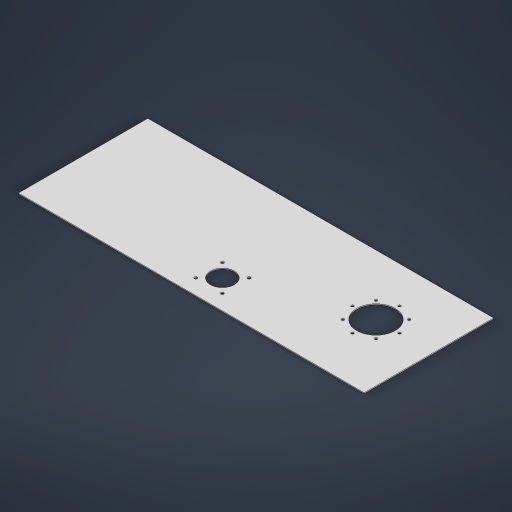
# Autodesk Inventor part: ElectronicsBoxLid
Saved by Autodesk Inventor 2024 (Build 280153000, 153)
## iProperties
Created: 2023-12-19
Part Number: ElectronicsBoxLid
Material: Generic
Document SubType Name: Modeling
Designer: avsar
Density: 1 g/cm^3
Appearance: Default
Author: avsar
Autodesk Inventor part; units mm, degrees
ref_plane "YZ Plane" through (0, 0, 0) normal (1, 0, 0) x (0, 1, 0)
ref_plane "XZ Plane" through (0, 0, 0) normal (0, 1, 0) x (-1, 0, 0)
ref_plane "XY Plane" through (0, 0, 0) normal (0, 0, 1) x (1, 0, 0)
sketch "Sketch1" plane through (0, 0, 0) normal (0, 1, 0) x (-1, 0, 0)
  line L0 (305.435, 114.3) -> (-305.435, 114.3)
  line L1 (-305.435, 114.3) -> (-305.435, -114.3)
  line L2 (-305.435, -114.3) -> (305.435, -114.3)
  line L3 (305.435, -114.3) -> (305.435, 114.3)
  line L4 (305.435, 114.3) -> (-305.435, -114.3) construction
  line L5 (-305.435, 114.3) -> (305.435, -114.3) construction
  point P0 (0, 0)
  dimension "d0" = 610.87
  dimension "d1" = 228.6
  constraints: 12 end point, 2 midpoint, 2 parallel, 1 horizontal, 1 perpendicular
  measures "d0" distance of L2.end L1.end
  measures "d1" distance of L1.end L0.end
extrude "Extrusion1" add sketch "Sketch1" along normal blind 1.5875
sketch "Sketch2" plane through (0, 1.5875, 0) normal (0, 1, 0) x (1, 0, 0)
  circle A0 centre (204, 8) radius 34
  circle A1 centre (204, 49.5) radius 2.25
  circle A2 centre (174.6551, 37.3449) radius 2.25
  circle A3 centre (162.5, 8) radius 2.25
  circle A4 centre (174.6551, -21.3449) radius 2.25
  circle A5 centre (204, -33.5) radius 2.25
  circle A6 centre (233.3449, -21.3449) radius 2.25
  circle A7 centre (245.5, 8) radius 2.25
  circle A8 centre (233.3449, 37.3449) radius 2.25
  point P0 (0, 0)
  dimension "d4" = 68
  dimension "d6" = 4.5
  dimension "d7" = 41.5
  dimension "d10" = 360
  dimension "d15" = 204
  dimension "d16" = 8
  constraints: 9 centre point, 1 vertical alignment, 17 other
  measures "d4" diameter of A0
  measures "d6" diameter of A1
  measures "d7" distance of A0.centre A1.centre
  measures "d15" horizontal distance of point (0, 0) A0.centre
  measures "d16" vertical distance of point (0, 0) A0.centre
extrude "Extrusion2" cut sketch "Sketch2" against normal blind 1.5875
sketch "Sketch3" plane through (0, 1.5875, 0) normal (0, 1, 0) x (1, 0, 0)
  circle A0 centre (4.6009, -64) radius 21
  circle A1 centre (204, 8) radius 34 construction
  circle A2 centre (204, 8) radius 106 construction
  circle A3 centre (-18.9691, -87.57) radius 2.55
  circle A4 centre (28.1709, -87.57) radius 2.55
  circle A5 centre (28.1709, -40.43) radius 2.55
  circle A6 centre (-18.9691, -40.43) radius 2.55
  line L0 (4.6009, -64) -> (204, 8) construction
  point P0 (0, 0)
  dimension "d17" = 42
  dimension "d18" = 212
  dimension "d20" = 72
  dimension "d21" = 5.1
  dimension "d22" = 23.57
  dimension "d23" = 23.57
  dimension "d26" = 360
  dimension "d30" = 212
  constraints: 6 centre point, 2 end point, 1 coincident, 9 other
  measures "d17" diameter of A0
  measures "d18" diameter of A2
  measures "d20" vertical distance of A1.centre L0.start
  measures "d21" diameter of A3
  measures "d22" horizontal distance of L0.start A3.centre
  measures "d23" horizontal distance of L0.start A3.centre
  measures "d30" distance of L0.start L0.end
extrude "Extrusion3" cut sketch "Sketch3" against normal through all
equation "\"d23\" = d22"
body "Solid1"
